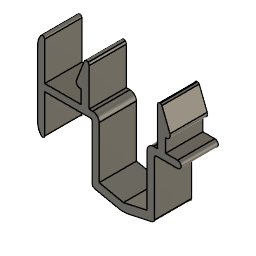
AdaptadorOXXO (Autodesk Fusion 360 design; units mm, degrees)
part number: 2025-12-28-15-28-43-770
Autodesk Fusion 360 part; units mm, degrees
sketch "Boceto1" plane through (0, 0, 0) normal (0, 1, 0) x (1, 0, 0)
  line L0 (0, 0) -> (0, -9.3) construction
  line L1 (0, -9.3) -> (0, -27.2)
  line L2 (0, -18.25) -> (38.3351, -18.25) construction
  line L3 (1.9, -19.2) -> (1.9, -29.5)
  arc A0 (0, -27.2) -> (0.8665, -29.847) centre (4.4763, -27.2) ccw
  arc A1 (0.8548, -29.8309) -> (1.9, -29.5) centre (1.325, -29.5) ccw
  line L4 (1.9, -19.2) -> (11.65, -19.2)
  line L5 (11.65, -19.2) -> (11.65, -22.8)
  line L6 (1.9, -17.3) -> (1.9, -7)
  arc A2 (0.8842, -6.7076) -> (0, -9.3) centre (4.2426, -9.3) ccw
  arc A3 (1.9, -7) -> (0.8842, -6.7076) centre (1.35, -7) ccw
  line L7 (1.9, -17.3) -> (14.1, -17.3)
  line L8 (14.6, -16.8) -> (14.6, -2.2063)
  line L9 (15.1929, -1.473) -> (21.5772, -0.1049)
  line L10 (24.4221, -0.1084) -> (30.709, -1.4718)
  line L11 (31.3, -2.2048) -> (31.3, -16.8)
  line L12 (31.8, -17.3) -> (37.5, -17.3)
  line L13 (37.5, -19.2) -> (34.3, -19.2)
  arc A4 (37.5, -19.2) -> (37.5, -17.3) centre (37.5, -18.25) ccw
  line L14 (13.8, -19.2) -> (13.8, -29.3)
  line L15 (12.5158, -29.7176) -> (10.3843, -24.1361)
  arc A5 (11.65, -22.8) -> (10.3843, -24.1361) centre (11.4728, -23.8997) ccw
  arc A6 (12.5158, -29.7176) -> (12.5233, -29.7366) centre (13.2164, -29.45) ccw
  arc A7 (13.5309, -29.9418) -> (13.8, -29.3) centre (12.9, -29.3) ccw
  arc A8 (12.5233, -29.7366) -> (13.5309, -29.9418) centre (13.0963, -29.4997) ccw
  line L16 (13.8, -19.2) -> (14.75, -19.2)
  line L17 (16.5, -17.45) -> (16.5, -3.5)
  line L18 (16.5, -3.5) -> (23, -2.1071)
  line L19 (23, -2.1071) -> (29.3055, -3.5)
  line L20 (29.3055, -3.5) -> (29.3055, -17.45)
  line L21 (31.0555, -19.2) -> (32.1, -19.2)
  line L22 (32.1, -19.2) -> (32.1, -29.5572)
  line L23 (34.3, -19.2) -> (34.3, -22.8)
  arc A9 (14.75, -19.2) -> (16.5, -17.45) centre (14.75, -17.45) ccw
  arc A10 (29.3055, -17.45) -> (31.0555, -19.2) centre (31.0555, -17.45) ccw
  arc A11 (14.1, -17.3) -> (14.6, -16.8) centre (14.1, -16.8) ccw
  arc A12 (31.3, -16.8) -> (31.8, -17.3) centre (31.8, -16.8) ccw
  line L24 (32.65, -30.1072) -> (32.8596, -30.1072)
  line L25 (33.3248, -29.7905) -> (35.4783, -24.3242)
  arc A13 (35.4783, -24.3242) -> (34.3, -22.8) centre (34.435, -23.9132) ccw
  arc A14 (32.1, -29.5572) -> (32.65, -30.1072) centre (32.65, -29.5572) ccw
  arc A15 (32.8596, -30.1072) -> (33.3248, -29.7905) centre (32.8596, -29.6072) ccw
  arc A16 (15.1929, -1.473) -> (14.6, -2.2063) centre (15.35, -2.2063) ccw
  arc A17 (31.3, -2.2048) -> (30.709, -1.4718) centre (30.55, -2.2048) ccw
  arc A18 (24.4221, -0.1084) -> (21.5772, -0.1049) centre (22.9915, -6.7051) ccw
  dimension "d1" = 0.75
  dimension "d2" = 0.9
  dimension "d3" = 0.62
  dimension "d4" = 1.75
  dimension "d5" = 0.5
  dimension "d6" = 0.55
  dimension "d7" = 0.5
  dimension "d8" = 0.75
  dimension "d9" = 6.75
  constraint coincident L0.start origin
  constraint vertical L0
  constraint parallel L0 L1
  constraint midpoint L1 L2.start
  constraint perpendicular L1 L2
  constraint coincident A0.end A1
  constraint tangent L1 A0
  constraint coincident A0 A1.start
  constraint perpendicular L1 L4
  constraint perpendicular L4 L5
  constraint perpendicular L2 L6
  constraint tangent L1 A2
  constraint perpendicular L6 L7
  constraint perpendicular L7 L8
  constraint perpendicular L7 L11
  constraint perpendicular L11 L12
  constraint perpendicular L11 L13
  constraint perpendicular L4 L14
  constraint tangent L15 A6
  constraint tangent L14 A7
  constraint tangent A7 A8
  constraint tangent A6 A8
  constraint perpendicular L14 L16
  constraint perpendicular L16 L17
  constraint parallel L9 L18
  constraint perpendicular L4 L20
  constraint perpendicular L17 L21
  constraint perpendicular L21 L22
  constraint perpendicular L13 L23
  constraint tangent L16 A9
  constraint tangent L17 A9
  constraint tangent L20 A10
  constraint tangent L21 A10
  constraint equal A9 A10
  constraint tangent L7 A11
  constraint tangent L8 A11
  constraint tangent L11 A12
  constraint tangent L12 A12
  constraint equal A11 A12
  constraint perpendicular L22 L24
  constraint tangent L25 A13
  constraint tangent L22 A14
  constraint tangent L24 A14
  constraint tangent L24 A15
  constraint tangent L25 A15
  constraint tangent L8 A16
  constraint tangent L9 A16
  constraint tangent L10 A17
  constraint tangent L11 A17
  constraint equal A16 A17
  constraint tangent L9 A18
  constraint tangent L10 A18
  measures "d1" radius of A6
  measures "d2" radius of A7
  measures "d3" radius of A8
  measures "d4" radius of A9
  measures "d5" radius of A11
  measures "d6" radius of A14
  measures "d7" radius of A15
  measures "d8" radius of A16
  measures "d9" radius of A18
extrude "Extruir1" add sketch "Boceto1" along normal blind 10
equation "L = 10 mm"
equation "d11 = L"
